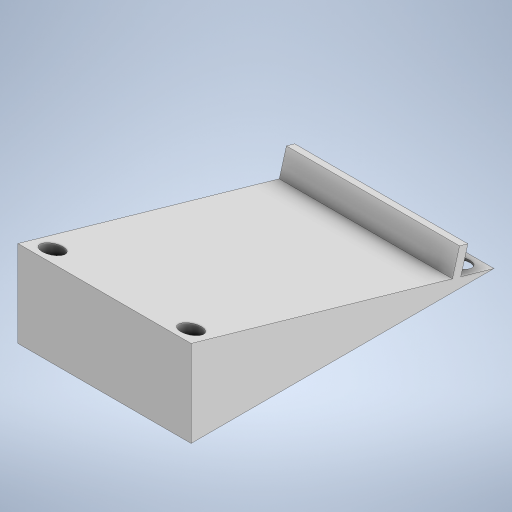
# Autodesk Inventor part: 1_mm_slant
Saved by Autodesk Inventor 2023.1 (Build 271208000, 208)
## iProperties
Created: 2023-05-29
Part Number: 1_mm_slant
Material: Generic
Document SubType Name: Modeling
Designer: Mansoor Lunawadi
Density: 1 g/cm^3
Appearance: Default
Author: Mansoor Lunawadi
Autodesk Inventor part; units mm, degrees
ref_plane "YZ Plane" through (0, 0, 0) normal (1, 0, 0) x (0, 1, 0)
ref_plane "XZ Plane" through (0, 0, 0) normal (0, 1, 0) x (-1, 0, 0)
ref_plane "XY Plane" through (0, 0, 0) normal (0, 0, 1) x (1, 0, 0)
sketch "Sketch1" plane through (0, 0, 0) normal (1, 0, 0) x (0, 1, 0)
  line L0 (0, 0) -> (10, 0)
  line L1 (0, 0) -> (0, -35)
  line L2 (0, -35) -> (10, 0)
  dimension "d0" = 10
  dimension "d1" = 35
  constraints: 6 end point, 1 horizontal, 1 vertical
  measures "d0" distance of L0.start L0.end
  measures "d1" distance of L0.start L1.end
extrude "Extrusion1" add sketch "Sketch1" along normal blind 20
sketch "Sketch2" plane through (0, 0, -35) normal (0, -1, 0) x (1, 0, 0)
  line L0 (0, 35) -> (20, 35) projected
  circle A0 centre (18, 33) radius 1.2
  line L1 (0, 35) -> (0, 0) projected
  circle A1 centre (2, 33) radius 1.2
  line L2 (20, 35) -> (20, 0) projected
  circle A2 centre (18, 2) radius 1.2
  circle A3 centre (2, 2) radius 1.2
  dimension "d6" = 2.4
  dimension "d8" = 2.4
  dimension "d12" = 2.4
  dimension "d13" = 2.4
  constraints: 4 centre point
  measures "d6" diameter of A0
  measures "d8" diameter of A1
  measures "d12" diameter of A2
  measures "d13" diameter of A3
extrude "Extrusion2" cut sketch "Sketch2" against normal through all
sketch "Sketch3" plane through (0, 10, 0) normal (0, 0.9615239, -0.2747211) x (1, 0, 0)
  line L0 (0, 2.7472) -> (0, 36.4005) projected
  line L1 (0, 36.4005) -> (0, 32.4005)
  line L2 (20, 2.7472) -> (20, 36.4005) projected
  line L3 (0, 32.4005) -> (20, 32.4005)
  line L4 (20, 32.4005) -> (20, 31.4005)
  line L5 (20, 31.4005) -> (0, 31.4005)
  line L6 (0, 31.4005) -> (0, 32.4005)
  dimension "d16" = 4
  dimension "d17" = 1
  constraints: 10 end point, 2 parallel, 2 point on line, 1 horizontal, 1 perpendicular
  measures "d16" distance of L0.end L1.end
  measures "d17" distance of L3.end L4.end
extrude "Extrusion3" add sketch "Sketch3" along normal blind 3
body "Solid1"
